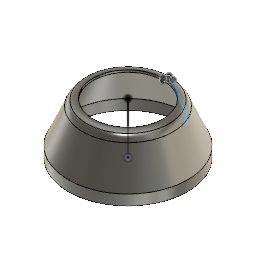
case (Autodesk Fusion 360 design; units mm, degrees)
Autodesk Fusion 360 part; units mm, degrees
sketch "Sketch1" plane through (0, 0, 0) normal (1, 0, 0) x (0, 1, 0)
  line L0 (85, 0) -> (85, 15)
  line L1 (85, 0) -> (82, 0)
  line L2 (82, 0) -> (82, 15)
  line L3 (0, 0) -> (0, 73)
  line L4 (50, 73) -> (50, 70)
  spline S0 degree 5 poles (50, 73) (50.4063, 73.0182) (51.2078, 73.0367) (52.3772, 73.0101) (53.8693, 72.8647) (55.6153, 72.487) (57.2317, 71.8962) (58.708, 71.0754) (60.0393, 70.0162) (61.2318, 68.7289) (62.2962, 67.2311) (63.0538, 65.8786) (63.5726, 64.7829) (63.8968, 64.0169) (64.0535, 63.625) knots 0 0 0 0 0 0 0.1 0.2 0.3 0.4 0.5 0.6 0.7 0.8 0.9 1 1 1 1 1 1
  line L5 (61.0535, 63.625) -> (82, 15)
  line L6 (51.9575, 70.0067) -> (50, 70)
  spline S1 degree 5 poles (50, 70) (50.3403, 70.0094) (51.0099, 70.0155) (51.9809, 69.9862) (53.2081, 69.8693) (54.6224, 69.5851) (55.9083, 69.1531) (57.0588, 68.5656) (58.0757, 67.825) (58.9739, 66.9493) (59.7664, 65.9537) (60.3249, 65.0717) (60.7043, 64.3654) (60.94, 63.8751) (61.0535, 63.625) knots 0 0 0 0 0 0 0.1 0.2 0.3 0.4 0.5 0.6 0.7 0.8 0.9 1 1 1 1 1 1
  line L7 (58.6014, 71.0627) -> (57.255, 68.3818)
  line L8 (55.9864, 69.2167) -> (58.5237, 67.5469)
  line L9 (64.0535, 63.625) -> (85, 15)
  line L10 (61.0535, 63.625) -> (64.0535, 63.625)
  point P0 (58.6014, 71.0627)
  point P1 (57.255, 68.3818)
  dimension "d21" = 3
  dimension "d23" = 15
  dimension "d24" = 85
  dimension "d38" = 73
  dimension "d41" = 3
  dimension "d46" = 3
  dimension "d48" = 3
  constraint perpendicular L1 L2
  constraint coincident L3.start origin
  constraint vertical L3
  constraint coincident P0 L7.start
  constraint coincident P1 L7.end
  constraint midpoint P1 L8
  constraint horizontal L10
  measures "d21" distance of L0.start L1.end
  measures "d23" distance of L1.end L2.end
  measures "d24" distance of L3.start L0.start
  measures "d38" distance of L3.start L3.end
  measures "d41" distance of L4.start L4.end
  measures "d46" distance of P0 P1
  measures "d48" distance of L5.start S0.end
sketch "Sketch2" plane through (0, 0, 0) normal (0, 0, 1) x (1, 0, 0)
revolve "Revolve3" add sketch "Sketch1" angle 360 about axis through (0, 0, 0) along (0, 0, 1)
